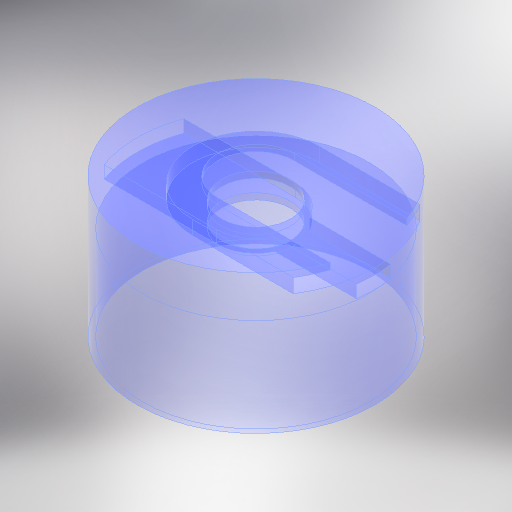
# Autodesk Inventor part: lens-holder_LIBS
Saved by Autodesk Inventor 2026 (Build 300175050, 175E)
## iProperties
Created: 2025-10-24
Part Number: lens-holder_LIBS
Material: ABS プラスチック
Document SubType Name: Modeling
Designer: jin20
Density: 1.06 g/cm^3
Appearance: クリア - 青
Author: jin20
Autodesk Inventor part; units mm, degrees
ref_plane "YZ Plane" through (0, 0, 0) normal (1, 0, 0) x (0, 1, 0)
ref_plane "XZ Plane" through (0, 0, 0) normal (0, 1, 0) x (-1, 0, 0)
ref_plane "XY Plane" through (0, 0, 0) normal (0, 0, 1) x (1, 0, 0)
sketch "スケッチ1" plane through (0, 0, 0) normal (0, 1, 0) x (-1, 0, 0)
  circle A0 centre (0, 0) radius 38
  dimension "d0" = 76
  constraints: 1 centre point, 1 coincident
  measures "d0" diameter of A0
extrude "押し出し1" add sketch "スケッチ1" along normal blind 36.5
sketch "スケッチ3" plane through (0, 36.5, 0) normal (0, 1, 0) x (1, 0, 0)
  circle A0 centre (0, 0) radius 20.25
  dimension "d6" = 40.5
  constraints: 1 centre point, 1 coincident
  measures "d6" diameter of A0
extrude "押し出し3" cut sketch "スケッチ3" against normal blind 6.5
sketch "スケッチ4" plane through (0, 36.5, 0) normal (0, 1, 0) x (1, 0, 0)
  circle A0 centre (0, 0) radius 20.25
  constraints: 1 centre point, 1 coincident
extrude "押し出し4" add sketch "スケッチ4" against normal blind 2
sketch "スケッチ6" plane through (0, 0, 0) normal (0, -1, 0) x (1, 0, 0)
  circle A0 centre (0, 0) radius 12.25
  dimension "d13" = 24.5
  constraints: 1 centre point, 1 coincident
  measures "d13" diameter of A0
extrude "押し出し5" cut sketch "スケッチ6" against normal through all
sketch "スケッチ7" plane through (0, 0, 0) normal (1, 0, 0) x (0, 1, 0)
  line L0 (34.5, -20.25) -> (34.5, 20.25) projected
  line L1 (30, 20.25) -> (30, -20.25) projected
  line L2 (34.5, 20.25) -> (30, 20.25)
  line L3 (30, 20.25) -> (30, -20.25)
  line L4 (30, -20.25) -> (34.5, -20.25)
  line L5 (34.5, -20.25) -> (34.5, 20.25)
  point P0 (0, 0)
  constraints: 8 end point, 2 parallel, 1 horizontal, 1 perpendicular
extrude "押し出し6" cut sketch "スケッチ7" along normal through all
sketch "スケッチ8" plane through (0, 0, 0) normal (1, 0, 0) x (0, 1, 0)
  line L0 (36.5, 12.25) -> (36.5, -12.25) projected
  line L1 (34.5, -12.25) -> (34.5, 12.25) projected
  line L2 (36.5, 12.25) -> (34.5, 12.25)
  line L3 (34.5, 12.25) -> (34.5, -12.25)
  line L4 (34.5, -12.25) -> (36.5, -12.25)
  line L5 (36.5, -12.25) -> (36.5, 12.25)
  point P0 (0, 0)
  constraints: 8 end point, 2 parallel, 1 horizontal, 1 perpendicular
extrude "押し出し7" cut sketch "スケッチ8" along normal through all
sketch "スケッチ10" plane through (0, 0, 0) normal (0, -1, 0) x (1, 0, 0)
  circle A0 centre (0, 0) radius 12.25
  constraints: 1 centre point, 1 coincident
extrude "押し出し9" add sketch "スケッチ10" against normal blind 30
sketch "スケッチ11" plane through (0, 0, 0) normal (0, -1, 0) x (1, 0, 0)
  circle A0 centre (0, 0) radius 11
  dimension "d25" = 22
  constraints: 1 centre point, 1 coincident
  measures "d25" diameter of A0
extrude "押し出し10" cut sketch "スケッチ11" against normal through all
sketch "スケッチ13" plane through (0, 0, 0) normal (0, 0, 1) x (1, 0, 0)
  line L0 (-11, 30) -> (11, 30) projected
  line L1 (0, 30) -> (0, 28) construction
  line L2 (0, 28) -> (-12.75, 28)
  line L3 (-12.75, 28) -> (-12.75, 24)
  line L4 (-12.75, 24) -> (0, 24)
  line L5 (0, 24) -> (0, 28)
  line L6 (0, -7.3) -> (0, 43.8) projected
  point P0 (0, 0)
  dimension "d29" = 2
  dimension "d30" = 12.75
  dimension "d31" = 4
  constraints: 10 end point, 2 parallel, 1 horizontal, 1 midpoint, 1 perpendicular, 1 vertical
  measures "d29" distance of L1.start L1.end
  measures "d30" distance of L4.end L3.end
  measures "d31" distance of L3.end L2.end
revolve "回転2" cut sketch "スケッチ13" angle 360 about axis through (0, -10, 0) along (0, -1, 0)
sketch "スケッチ14" plane through (0, 0, 0) normal (1, 0, 0) x (0, 1, 0)
  line L0 (28, 12.75) -> (24, 12.75) projected
  line L1 (28, -12.75) -> (24, -12.75) projected
  line L2 (24, 12.75) -> (28, 12.75)
  line L3 (28, 12.75) -> (28, -12.75)
  line L4 (28, -12.75) -> (24, -12.75)
  line L5 (24, -12.75) -> (24, 12.75)
  point P0 (0, 0)
  constraints: 8 end point, 2 parallel, 2 point on line, 1 horizontal, 1 perpendicular
extrude "押し出し11" cut sketch "スケッチ14" against normal through all
sketch "スケッチ15" plane through (0, 0, 0) normal (1, 0, 0) x (0, 1, 0)
  line L0 (24, 0) -> (24, -5.5)
  line L1 (24, -5.5) -> (28, -5.5)
  line L2 (28, -5.5) -> (28, 0)
  line L3 (24, 0) -> (24, 5.5)
  line L4 (24, 5.5) -> (28, 5.5)
  line L5 (28, 5.5) -> (28, 0)
  point P0 (0, 0)
  dimension "d35" = 4
  dimension "d36" = 5.5
  constraints: 12 end point, 1 parallel
  measures "d35" distance of L1.end L0.end
  measures "d36" distance of L0.end L0.start
extrude "押し出し12" cut sketch "スケッチ15" along normal through all
sketch "スケッチ16" plane through (0, 0, 0) normal (0, -1, 0) x (1, 0, 0)
  circle A0 centre (0, 0) radius 38
  constraints: 1 centre point, 1 coincident
extrude "押し出し13" add sketch "スケッチ16" along normal blind 8
sketch "スケッチ17" plane through (0, -8, 0) normal (0, -1, 0) x (1, 0, 0)
  circle A0 centre (0, 0) radius 11
  constraints: 1 centre point, 1 coincident
extrude "押し出し14" cut sketch "スケッチ17" against normal through all
sketch "スケッチ19" plane through (0, -8, 0) normal (0, -1, 0) x (1, 0, 0)
  circle A0 centre (0, 0) radius 36.25
  dimension "d44" = 72.5
  constraints: 1 centre point, 1 coincident
  measures "d44" diameter of A0
extrude "押し出し15" cut sketch "スケッチ19" against normal blind 30
